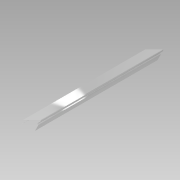
# Autodesk Inventor part: MGN12
Saved by Autodesk Inventor 2016 (Build 200138000, 138)
## iProperties
Created: 2017-05-18
Part Number: MGN12
Material: Generic
Document SubType Name: Modeling
Designer: 31745
Density: 1 g/cm^3
Appearance: Aluminum - Dark
Author: 31745
Autodesk Inventor part; units mm, degrees
ref_plane "YZ Plane" through (0, 0, 0) normal (1, 0, 0) x (0, 1, 0)
ref_plane "XZ Plane" through (0, 0, 0) normal (0, 1, 0) x (-1, 0, 0)
ref_plane "XY Plane" through (0, 0, 0) normal (0, 0, 1) x (1, 0, 0)
sketch "Sketch1" plane through (0, 0, 0) normal (0, 0, 1) x (1, 0, 0)
  line L0 (0, 0) -> (12, 0)
  line L1 (12, 0) -> (12, 8)
  line L2 (12, 8) -> (0, 8)
  line L3 (0, 8) -> (0, 0)
  line L4 (12, 8) -> (12, 4.75)
  line L5 (12, 4.75) -> (11, 4.75)
  line L6 (11, 4.75) -> (11, 5.75)
  line L7 (11, 5.75) -> (12, 5.75)
  line L8 (0, 5.75) -> (1, 5.75)
  line L9 (1, 5.75) -> (1, 4.75)
  line L10 (1, 4.75) -> (0, 4.75)
  dimension "d0" = 8
  dimension "d1" = 12
  dimension "d2" = 3.25
  dimension "d3" = 2.25
  dimension "d4" = 1
  dimension "d5" = 1
  constraints: 22 end point, 4 perpendicular, 4 point on line, 3 horizontal, 2 horizontal alignment, 2 parallel, 1 vertical
  measures "d0" distance of L0.end L1.end
  measures "d1" distance of L1.end L2.end
  measures "d2" distance between parallel lines of L2 L5
  measures "d3" distance between parallel lines of L2 L7
  measures "d4" distance between parallel lines of L1 L6
  measures "d5" distance of L8.start L8.end
extrude "Extrusion1" add sketch "Sketch1" against normal blind 196.85 contours L3 L10 L9 L8 L2 L1 L7 L6 L5 L0
chamfer "Chamfer1" distance 0.5 angle 45 4 edges at (12, 5.75, -98.425) (12, 4.75, -98.425) (0, 5.75, -98.425) (0, 4.75, -98.425)
chamfer "Chamfer2" distance 0.375 angle 45 2 edges at (12, 8, -98.425) (0, 8, -98.425)
equation "\"d4\" = d5"
body "Solid1"
